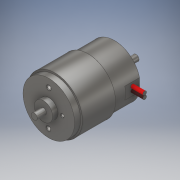
# Autodesk Inventor part: モータ RZ-735VA
Saved by Autodesk Inventor 2019 (Build 230136000, 136)
## iProperties
Created: 2020-10-24
Part Number: モータ RZ-735VA
Material: ステンレス鋼
Document SubType Name: Modeling
Designer: Toshihito
Density: 8 g/cm^3
Appearance: 半つや出し
Author: Toshihito
Autodesk Inventor part; units mm, degrees
ref_plane "YZ Plane" through (0, 0, 0) normal (1, 0, 0) x (0, 1, 0)
ref_plane "XZ Plane" through (0, 0, 0) normal (0, 1, 0) x (-1, 0, 0)
ref_plane "XY Plane" through (0, 0, 0) normal (0, 0, 1) x (1, 0, 0)
sketch "スケッチ1" plane through (0, 0, 0) normal (0, 0, 1) x (1, 0, 0)
  circle A0 centre (0, 0) radius 2.5
  dimension "d0" = 5
  constraints: 1 centre point, 1 coincident
  measures "d0" diameter of A0
extrude "押し出し1" add sketch "スケッチ1" along normal blind 7.5
sketch "スケッチ2" plane through (0, 0, 0) normal (0, 0, -1) x (-1, 0, 0)
  circle A0 centre (0, 0) radius 7.5
  dimension "d3" = 15
  constraints: 1 centre point, 1 coincident
  measures "d3" diameter of A0
extrude "押し出し2" add sketch "スケッチ2" along normal blind 4.4
sketch "スケッチ3" plane through (0, 0, -4.4) normal (0, 0, -1) x (-1, 0, 0)
  circle A0 centre (0, 0) radius 7.5 projected
  circle A1 centre (0, 0) radius 21.05
  dimension "d6" = 42.1
  constraints: 1 centre point, 1 coincident
  measures "d6" diameter of A1
extrude "押し出し3" add sketch "スケッチ3" along normal blind 4.9
sketch "スケッチ4" plane through (0, 0, -9.3) normal (0, 0, -1) x (-1, 0, 0)
  circle A0 centre (0, 0) radius 22.5
  dimension "d9" = 45
  constraints: 1 centre point, 1 coincident
  measures "d9" diameter of A0
extrude "押し出し4" add sketch "スケッチ4" along normal blind 27
sketch "スケッチ5" plane through (0, 0, -36.3) normal (0, 0, -1) x (-1, 0, 0)
  circle A0 centre (0, 0) radius 21.05
  dimension "d12" = 42.1
  constraints: 1 centre point, 1 coincident
  measures "d12" diameter of A0
extrude "押し出し5" add sketch "スケッチ5" along normal blind 21.6
sketch "スケッチ6" plane through (0, 0, -57.9) normal (0, 0, -1) x (-1, 0, 0)
  circle A0 centre (0, 0) radius 7.5
  dimension "d15" = 15
  constraints: 1 centre point, 1 coincident
  measures "d15" diameter of A0
extrude "押し出し6" add sketch "スケッチ6" along normal blind 4.3
sketch "スケッチ7" plane through (0, 0, -62.2) normal (0, 0, -1) x (-1, 0, 0)
  circle A0 centre (0, 0) radius 2.5
  dimension "d18" = 5
  constraints: 1 centre point, 1 coincident
  measures "d18" diameter of A0
extrude "押し出し7" add sketch "スケッチ7" along normal blind 13.3
sketch "スケッチ8" plane through (0, 0, -4.4) normal (0, 0, 1) x (1, 0, 0)
  point P0 (0, 0)
  point P1 (0.0124, 14.5)
  point P2 (-0.3227, -14.5)
  dimension "d35" = 14.5
  dimension "d36" = 14.5
  measures "d35" distance of point (0.012, 14.5) point (0, 0)
  measures "d36" vertical distance of point (0, 0) point (-0.323, -14.5)
hole "穴1" at (0.0124, 14.5, -4.4) at (-0.3227, -14.5, -4.4) direction (0, 0, -1) diameter 4 depth 0.7 tip angle 118
sketch "スケッチ9" plane through (0, 0, -4.4) normal (0, 0, 1) x (1, 0, 0)
  point P0 (0, 0)
  point P1 (11, 0.2443)
  dimension "d37" = 11
  measures "d37" horizontal distance of point (11, 0.244) point (0, 0)
hole "穴2" at (11, 0.2443, -4.4) direction (0, 0, -1) diameter 3 depth 0.7 tip angle 118
sketch "スケッチ10" plane through (0, 0, -57.9) normal (0, 0, -1) x (-1, 0, 0)
  circle A0 centre (0, 0) radius 21.05 projected
  arc A1 (-20.4476, 5) -> (-20.4476, -5) centre (0, 0) ccw
  line L0 (-20.4476, -5) -> (-20.4476, 5)
  dimension "d38" = 5
  dimension "d39" = 5
  constraints: 4 point on circle, 2 end point, 1 centre point, 1 coincident
  measures "d38" vertical distance of point (0, 0) L0.start
  measures "d39" vertical distance of point (0, 0) L0.end
extrude "押し出し8" cut sketch "スケッチ10" against normal blind 12 contours L0 A0 picked at (-20.626, 0.5603)
sketch "スケッチ11" plane through (20.4476, -5, -57.9) normal (1, 0, 0) x (0, 0, -1)
  circle A0 centre (-5.7655, 6.983) radius 1.5
  circle A1 centre (-5.7655, 3.8896) radius 1.5
  point P0 (-57.9, 5)
  dimension "d42" = 3
  dimension "d43" = 3
  constraints: 2 centre point
  measures "d42" diameter of A0
  measures "d43" diameter of A1
extrude "押し出し9" add sketch "スケッチ11" along normal blind 10
equation "\"d36\" = d35"
equation "\"d39\" = d38"
